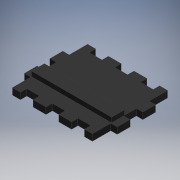
# Autodesk Inventor part: front
Saved by Autodesk Inventor 2019 (Build 230136000, 136)
## iProperties
Created: 2018-06-06
Part Number: front
Material: PBT Plastic Black
Document SubType Name: Modeling
Designer: stra92745
Density: 1.31 g/cm^3
Appearance: Smooth - White
Author: stra92745
Autodesk Inventor part; units mm, degrees
ref_plane "YZ Plane" through (0, 0, 0) normal (1, 0, 0) x (0, 1, 0)
ref_plane "XZ Plane" through (0, 0, 0) normal (0, 1, 0) x (-1, 0, 0)
ref_plane "XY Plane" through (0, 0, 0) normal (0, 0, 1) x (1, 0, 0)
sketch "Sketch1" plane through (0, 0, 0) normal (0, 1, 0) x (-1, 0, 0)
  line L0 (0, 0) -> (-58, 0)
  line L1 (-58, 0) -> (-58, -47)
  line L2 (-58, -47) -> (0, -47)
  line L3 (0, -47) -> (0, 0)
  dimension "d0" = 58
  dimension "d1" = 47
  constraints: 8 end point, 2 parallel, 1 horizontal, 1 perpendicular
  measures "d0" distance of L2.end L1.end
  measures "d1" distance of L1.end L0.end
extrude "Extrusion1" add sketch "Sketch1" along normal blind 4
sketch "Sketch2" plane through (0, 4, 0) normal (0, 1, 0) x (1, 0, 0)
  line L0 (58, 47) -> (0, 47) projected
  line L1 (0, 47) -> (0, 0) projected
  line L2 (0, 0) -> (58, 0) projected
  line L3 (58, 0) -> (58, 47) projected
  line L4 (4, 43) -> (54, 43)
  line L5 (54, 43) -> (54, 4)
  line L6 (54, 4) -> (4, 4)
  line L7 (4, 4) -> (4, 43)
  line L8 (4, 47) -> (4, 35.5)
  line L9 (4, 35.5) -> (0, 35.5)
  line L10 (0, 47) -> (4, 47)
  line L11 (0, 35.5) -> (0, 47)
  line L12 (0, 23.5) -> (58, 23.5) construction
  line L13 (4, 27.5) -> (0, 27.5)
  line L14 (0, 27.5) -> (0, 23.5)
  line L15 (4, 27.5) -> (4, 23.5)
  line L16 (29, 23.5) -> (29, 47) construction
  line L17 (9, 47) -> (9, 43)
  line L18 (9, 43) -> (17, 43)
  line L19 (17, 43) -> (17, 47)
  line L20 (9, 47) -> (17, 47)
  line L21 (25, 47) -> (25, 43)
  line L22 (29, 43) -> (25, 43)
  line L23 (25, 47) -> (29, 47)
  line L24 (54, 47) -> (54, 35.5)
  line L25 (54, 35.5) -> (58, 35.5)
  line L26 (58, 47) -> (54, 47)
  line L27 (58, 35.5) -> (58, 47)
  line L28 (54, 27.5) -> (58, 27.5)
  line L29 (58, 27.5) -> (58, 23.5)
  line L30 (54, 27.5) -> (54, 23.5)
  line L31 (49, 47) -> (49, 43)
  line L32 (49, 43) -> (41, 43)
  line L33 (41, 43) -> (41, 47)
  line L34 (49, 47) -> (41, 47)
  line L35 (33, 47) -> (33, 43)
  line L36 (29, 43) -> (33, 43)
  line L37 (33, 47) -> (29, 47)
  line L38 (58, 0) -> (0, 0)
  line L39 (4, 4) -> (54, 4)
  line L40 (4, 0) -> (4, 11.5)
  line L41 (4, 11.5) -> (0, 11.5)
  line L42 (0, 0) -> (4, 0)
  line L43 (0, 11.5) -> (0, 0)
  line L44 (4, 19.5) -> (0, 19.5)
  line L45 (0, 19.5) -> (0, 23.5)
  line L46 (4, 19.5) -> (4, 23.5)
  line L47 (29, 23.5) -> (29, 0) construction
  line L48 (9, 0) -> (9, 4)
  line L49 (9, 4) -> (17, 4)
  line L50 (17, 4) -> (17, 0)
  line L51 (9, 0) -> (17, 0)
  line L52 (25, 0) -> (25, 4)
  line L53 (29, 4) -> (25, 4)
  line L54 (25, 0) -> (29, 0)
  line L55 (58, 19.5) -> (58, 23.5)
  line L56 (54, 19.5) -> (54, 23.5)
  line L57 (54, 11.5) -> (58, 11.5)
  line L58 (58, 11.5) -> (58, 0)
  line L59 (58, 0) -> (54, 0)
  line L60 (29, 4) -> (33, 4)
  line L61 (33, 0) -> (33, 4)
  line L62 (33, 0) -> (29, 0)
  line L63 (54, 19.5) -> (58, 19.5)
  line L64 (54, 0) -> (54, 11.5)
  line L65 (49, 4) -> (41, 4)
  line L66 (41, 4) -> (41, 0)
  line L67 (49, 0) -> (49, 4)
  line L68 (49, 0) -> (41, 0)
  dimension "d8" = 4
  dimension "d11" = 8
  dimension "d12" = 8
  dimension "d13" = 4
  dimension "d16" = 4
  dimension "d17" = 8
  constraints: 130 end point, 36 symmetric about line, 21 point on line, 7 midpoint, 5 collinear, 5 perpendicular, 2 vertical, 3 other
  measures "d8" distance between parallel lines of L0 L4
  measures "d11" distance of L17.end L18.end
  measures "d12" distance between parallel lines of L21 L19
  measures "d13" distance between parallel lines of L16 L21
  measures "d16" distance between parallel lines of L12 L13
  measures "d17" distance between parallel lines of L13 L9
extrude "Extrusion2" cut sketch "Sketch2" against normal up to surface (4 mm away) contours L3 L25 L5 L24 L0 | L31 L4 L33 L0 | L3 L63 L5 L28 | L35 L4 L21 L0 | L3 L2 L64 L5 L57 | L19 L4 L17 L0 | L2 L66 L6 L67 | L8 L7 L9 L1 L0 | L2 L52 L6 L61 | L13 L7 L44 L1 | L2 L48 L6 L50 | L41 L7 L40 L2 L1
sketch "Sketch3" plane through (0, 4, 0) normal (0, 1, 0) x (1, 0, 0)
  line L0 (4, 11.5) -> (4, 0) projected
  line L1 (4, 12) -> (54, 12)
  line L2 (54, 12) -> (54, 20)
  line L3 (54, 20) -> (4, 20)
  line L4 (4, 20) -> (4, 12)
  line L5 (9, 4) -> (17, 4) projected
  point P0 (0, 0)
  dimension "d18" = 8
  dimension "d19" = 8
  constraints: 8 end point, 2 parallel, 1 horizontal, 1 perpendicular, 1 point on line
  measures "d18" distance between parallel lines of L5 L1
  measures "d19" distance between parallel lines of L1 L3
extrude "Extrusion3" add sketch "Sketch3" along normal blind 3
body "Solid1"
